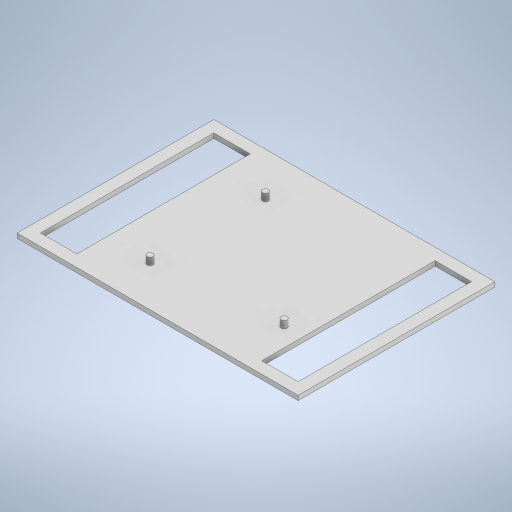
# Autodesk Inventor part: gora
Saved by Autodesk Inventor 2024 (Build 280153020, 153B)
## iProperties
Created: 2025-01-23
Part Number: gora
Material: Ogólny
Document SubType Name: Modeling
Designer: jakub
Density: 1 g/cm^3
Appearance: Domyślna
Author: jakub
Autodesk Inventor part; units mm, degrees
ref_plane "YZ Plane" through (0, 0, 0) normal (1, 0, 0) x (0, 1, 0)
ref_plane "XZ Plane" through (0, 0, 0) normal (0, 1, 0) x (-1, 0, 0)
ref_plane "XY Plane" through (0, 0, 0) normal (0, 0, 1) x (1, 0, 0)
sketch "Szkic1" plane through (0, 0, 0) normal (0, 1, 0) x (-1, 0, 0)
  line L0 (-60, 42.2624) -> (60, 42.2624)
  line L1 (60, 42.2624) -> (60, -41.7376)
  line L2 (60, -41.7376) -> (-60, -41.7376)
  line L3 (-60, -41.7376) -> (-60, 42.2624)
  line L4 (-34.5, 26.7624) -> (34.5, 26.7624)
  line L5 (34.5, 26.7624) -> (34.5, -26.2376)
  line L6 (34.5, -26.2376) -> (-34.5, -26.2376)
  line L7 (-34.5, -26.2376) -> (-34.5, 26.7624)
  line L8 (39.5, 37.2624) -> (55, 37.2624)
  line L9 (55, 37.2624) -> (55, -36.7376)
  line L10 (55, -36.7376) -> (39.5, -36.7376)
  line L11 (39.5, -36.7376) -> (39.5, 37.2624)
  line L12 (39.5, 37.2624) -> (55, -36.7376) construction
  line L13 (55, 37.2624) -> (39.5, -36.7376) construction
  line L14 (-39.5, 37.2624) -> (-55, 37.2624)
  line L15 (-55, 37.2624) -> (-55, -36.7376)
  line L16 (-55, -36.7376) -> (-39.5, -36.7376)
  line L17 (-39.5, -36.7376) -> (-39.5, 37.2624)
  line L18 (-39.5, 37.2624) -> (-55, -36.7376) construction
  line L19 (-55, 37.2624) -> (-39.5, -36.7376) construction
  circle A0 centre (19.5, -23.2376) radius 1.3
  line L20 (0, 0) -> (11.1545, 0)
  circle A1 centre (20.5, 23.7624) radius 1.3
  circle A2 centre (-31.5, 18.7624) radius 1.3
  circle A3 centre (20.5, 23.7624) radius 1.3
  circle A4 centre (19.5, -23.2376) radius 1.3
  circle A5 centre (-31.5, 18.7624) radius 1.3
  point P0 (47.25, 0.2624)
  dimension "d0" = 120
  dimension "d1" = 84
  dimension "d4" = 69
  dimension "d5" = 53
  dimension "d8" = 5
  dimension "d9" = 5
  dimension "d13" = 2.6
  dimension "d14" = 3
  dimension "d15" = 15
  dimension "d16" = 15.5
  dimension "d17" = 15.5
  dimension "d18" = 25.5
  dimension "d19" = 5
  dimension "d20" = 5
  dimension "d23" = 2.6
  dimension "d24" = 3
  dimension "d25" = 14
  dimension "d28" = 2.6
  constraints: 42 end point, 6 centre point, 6 parallel, 4 horizontal, 3 coincident, 3 concentric, 3 perpendicular, 2 midpoint
  measures "d0" distance of L1.end L2.end
  measures "d1" distance of L0.end L1.end
  measures "d4" distance of L5.end L6.end
  measures "d5" distance of L4.end L5.end
  measures "d8" distance between parallel lines of L2 L10
  measures "d9" distance between parallel lines of L0 L8
  measures "d13" diameter of A0
  measures "d14" distance from line of L6 A0.centre
  measures "d15" distance from line of L5 A0.centre
  measures "d16" distance between parallel lines of L0 L4
  measures "d17" distance between parallel lines of L2 L6
  measures "d18" distance between parallel lines of L1 L5
  measures "d19" distance between parallel lines of L7 L17
  measures "d20" distance between parallel lines of L3 L15
  measures "d23" diameter of A1
  measures "d24" distance from line of L4 A1.centre
  measures "d25" distance from line of L5 A1.centre
  measures "d28" diameter of A2
extrude "Wyciągnięcie proste1" add sketch "Szkic1" along normal blind 2 contours L0 L1 L2 L3 | L4 L5 L6 L7
sketch "Szkic3" plane through (0, 0, 0) normal (0, -1, 0) x (1, 0, 0)
  circle A0 centre (-20.5, 23.7624) radius 1.3
  circle A1 centre (31.5, 18.7624) radius 1.3 projected
  circle A2 centre (-19.5, -23.2376) radius 1.3 projected
  circle A3 centre (-19.5, -23.2376) radius 1.3
  circle A4 centre (-20.5, 25.0124) radius 1.3
  line L0 (31.5, 18.7624) -> (31.5, 19.7624)
  circle A5 centre (31.5, 19.7624) radius 1.3
  point P0 (0, 0)
  dimension "d31" = 2.6
  dimension "d32" = 48.25
  dimension "d36" = 1
  constraints: 4 centre point, 3 coincident, 2 end point, 1 vertical
  measures "d31" diameter of A4
  measures "d32" vertical distance of A3.centre A4.centre
  measures "d36" distance of L0.start L0.end
extrude "Wyciągnięcie proste2" add sketch "Szkic3" against normal blind 5 contours A4 A0 | A0 A4 | A5 A1 | A1 A5 | A2 picked at (-20.4486, 24.1655) picked at (-20.5582, 25.8863) picked at (31.399, 19.5171) picked at (31.6684, 20.3785)
sketch "Szkic4" plane through (0, 0, 0) normal (0, -1, 0) x (1, 0, 0)
  arc A0 (-21.6399, 24.3874) -> (-19.3601, 24.3874) centre (-20.5, 23.7624) ccw projected
  circle A1 centre (-20.5, 23.7624) radius 1.3
  arc A2 (30.3, 19.2624) -> (32.7, 19.2624) centre (31.5, 18.7624) ccw projected
  circle A3 centre (31.5, 18.7624) radius 1.3
  point P0 (0, 0)
  point P1 (32.7, 19.2624)
  constraints: 2 centre point, 2 coincident
extrude "Wyciągnięcie proste3" add sketch "Szkic4" against normal blind 2
